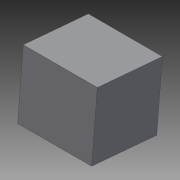
# Autodesk Inventor part: Part1
Saved by Autodesk Inventor 2014 SP2 (Build 180246200, 246)
## iProperties
Created: 2014-12-30
Part Number: Part1
Material: 一般
Document SubType Name: Modeling
Designer: hiratayuya
Density: 1 g/cm^3
Appearance: 既定
Author: hiratayuya
Autodesk Inventor part; units mm, degrees
ref_plane "YZ Plane" through (0, 0, 0) normal (1, 0, 0) x (0, 1, 0)
ref_plane "XZ Plane" through (0, 0, 0) normal (0, 1, 0) x (-1, 0, 0)
ref_plane "XY Plane" through (0, 0, 0) normal (0, 0, 1) x (1, 0, 0)
sketch "スケッチ1" plane through (0, 0, 0) normal (0, 1, 0) x (-1, 0, 0)
  line L0 (-7.5, -10) -> (7.5, -10)
  line L1 (7.5, -10) -> (7.5, 10)
  line L2 (7.5, 10) -> (-7.5, 10)
  line L3 (-7.5, 10) -> (-7.5, -10)
  line L4 (-7.5, -10) -> (7.5, 10) construction
  line L5 (7.5, -10) -> (-7.5, 10) construction
  line L6 (-7.5, 10) -> (7.5, 10)
  line L7 (7.5, 10) -> (7.5, 4)
  line L8 (7.5, 4) -> (-7.5, 4)
  line L9 (-7.5, 4) -> (-7.5, 10)
  line L10 (-7.5, -10) -> (7.5, -10)
  line L11 (7.5, -10) -> (7.5, -4)
  line L12 (7.5, -4) -> (-7.5, -4)
  line L13 (-7.5, -4) -> (-7.5, -10)
  point P0 (0, 0)
  dimension "d0" = 15
  dimension "d1" = 20
  dimension "d2" = 6
  dimension "d3" = 6
  constraints: 28 end point, 6 parallel, 3 horizontal, 3 perpendicular, 2 midpoint, 2 point on line
  measures "d0" distance of L1.end L2.end
  measures "d1" distance of L0.end L1.end
  measures "d2" distance between parallel lines of L8 L6
  measures "d3" distance between parallel lines of L10 L12
extrude "押し出し1" add sketch "スケッチ1" along normal blind 6 contours L3 L12 L1 L0 | L3 L2 L1 L8
sketch "スケッチ2" plane through (0, 6, 0) normal (0, 1, 0) x (1, 0, 0)
  line L0 (7.5, 10) -> (-7.5, 10) projected
  line L1 (-7.5, 10) -> (-7.5, 4) projected
  line L2 (-7.5, 4) -> (7.5, 4) projected
  line L3 (7.5, 4) -> (7.5, 10) projected
  line L4 (-7.5, -5.5) -> (7.5, -5.5)
  line L5 (7.5, -5.5) -> (7.5, 5.5)
  line L6 (7.5, 5.5) -> (-7.5, 5.5)
  line L7 (-7.5, 5.5) -> (-7.5, -5.5)
  line L8 (-7.5, -5.5) -> (7.5, 5.5) construction
  line L9 (7.5, -5.5) -> (-7.5, 5.5) construction
  point P0 (0, 0)
  dimension "d6" = 11
  constraints: 12 end point, 2 midpoint, 2 parallel, 1 horizontal, 1 perpendicular, 1 point on line
  measures "d6" distance between parallel lines of L4 L6
extrude "押し出し2" add sketch "スケッチ2" along normal blind 20 contours L3 L2 L1 L6 | L5 L4 L7 L2
sketch "スケッチ3" plane through (7.5, 0, -4) normal (1, 0, 0) x (0, 0, -1)
  line L0 (1.5, 6) -> (1.5, 26) projected
  line L1 (-9.5, 26) -> (1.5, 26) projected
  line L2 (-9.5, 26) -> (1.5, 25.0376)
  point P0 (-4, 0)
  dimension "d9" = 5
  constraints: 2 end point, 1 point on line
  measures "d9" angle of L1 L2
extrude "押し出し3" cut sketch "スケッチ3" against normal blind 20
sketch "スケッチ4" plane through (-7.5, 26, 5.5) normal (0, 0.9961947, -0.0871557) x (1, 0, 0)
  line L0 (0, 0) -> (0, 11.042) projected
  line L1 (0, 0) -> (15, 0) projected
  line L2 (15, 11.042) -> (15, 0) projected
  line L3 (0, 11.042) -> (15, 11.042) projected
  line L4 (-2, 13.042) -> (17, 13.042)
  line L5 (17, 13.042) -> (17, -2)
  line L6 (17, -2) -> (-2, -2)
  line L7 (-2, -2) -> (-2, 13.042)
  point P0 (7.5, 7.7451)
  dimension "d12" = 2
  dimension "d13" = 2
  dimension "d14" = 2
  dimension "d15" = 2
  constraints: 8 end point, 2 parallel, 1 horizontal, 1 perpendicular
  measures "d12" distance between parallel lines of L4 L3
  measures "d13" distance between parallel lines of L6 L1
  measures "d14" distance between parallel lines of L5 L2
  measures "d15" distance between parallel lines of L0 L7
extrude "押し出し4" add sketch "スケッチ4" along normal blind 15 contours L0 L3 L2 L1 | L4 L5 L6 L7
sketch "スケッチ5" plane through (9.5, 24.8633, -7.4924) normal (0, -0.0871557, -0.9961947) x (-1, 0, 0)
  line L0 (19, 0) -> (0, 0) projected
  line L1 (11.6915, 7.5253) -> (11.6915, 2.7045)
  line L2 (11.6915, 2.7045) -> (7.6915, 2.7045)
  line L3 (7.6915, 2.7045) -> (7.6915, 7.5253)
  line L4 (9.6915, 7.5253) -> (11.6915, 2.7045) construction
  line L5 (9.6915, 7.5253) -> (7.6915, 2.7045) construction
  line L6 (7.6915, 7.5253) -> (11.6915, 7.5253)
  line L7 (11.6915, 5.1149) -> (13.1915, 5.1149)
  line L8 (13.1915, 5.1149) -> (13.1915, 1.1149)
  line L9 (13.1915, 1.1149) -> (11.6915, 1.1149)
  line L10 (11.6915, 1.1149) -> (11.6915, 5.1149)
  line L11 (7.6915, 5.1149) -> (6.1915, 5.1149)
  line L12 (6.1915, 5.1149) -> (6.1915, 1.1149)
  line L13 (6.1915, 1.1149) -> (7.6915, 1.1149)
  line L14 (7.6915, 1.1149) -> (7.6915, 5.1149)
  line L15 (11.6915, 7.5253) -> (14.6915, 7.5253)
  line L16 (14.6915, 7.5253) -> (14.6915, 10.5253)
  line L17 (14.6915, 10.5253) -> (11.6915, 10.5253)
  line L18 (11.6915, 10.5253) -> (11.6915, 7.5253)
  line L19 (7.6915, 7.5253) -> (4.6915, 7.5253)
  line L20 (4.6915, 7.5253) -> (4.6915, 10.5253)
  line L21 (4.6915, 10.5253) -> (7.6915, 10.5253)
  line L22 (7.6915, 10.5253) -> (7.6915, 7.5253)
  point P0 (9.5, -25.4217)
  dimension "d18" = 4
  dimension "d19" = 1.5
  dimension "d20" = 4
  dimension "d21" = 1.5
  dimension "d22" = 3
  dimension "d23" = 3
  dimension "d24" = 3
  dimension "d25" = 2.7045
  constraints: 44 end point, 9 parallel, 4 horizontal, 4 perpendicular, 3 midpoint, 2 point on line
  measures "d18" distance of L3.end L1.start
  measures "d19" distance of L7.start L7.end
  measures "d20" distance of L7.end L8.end
  measures "d21" distance of L13.end L12.end
  measures "d22" distance of L17.end L16.end
  measures "d23" distance of L15.end L16.end
  measures "d24" distance of L20.end L21.end
  measures "d25" distance between parallel lines of L0 L2
extrude "押し出し5" cut sketch "スケッチ5" against normal blind 1
sketch "スケッチ6" plane through (7.5, 0, 10) normal (1, 0, 0) x (0, 0, -1)
  line L0 (4.5, 6) -> (4.5, 26) projected
  line L1 (0, 6) -> (4.5, 6) projected
  line L2 (0, 0) -> (0, 6) projected
  line L3 (0, 0) -> (6, 0) projected
  line L4 (6, 0) -> (6, 6) projected
  line L5 (6, 6) -> (14, 6) projected
  line L6 (14, 0) -> (14, 6) projected
  line L7 (14, 0) -> (20, 0) projected
  line L8 (20, 0) -> (20, 6) projected
  line L9 (15.5, 6) -> (20, 6) projected
  line L10 (15.5, 6) -> (15.5, 25.0376) projected
  line L11 (15.5, 25.0376) -> (4.5, 25.0376)
  point P0 (10, 0)
  constraints: 2 end point, 1 perpendicular, 1 point on line
extrude "押し出し6" cut sketch "スケッチ6" against normal blind 100
sketch "スケッチ7" plane through (-7.5, 25.0376, 5.5) normal (-1, 0, 0) x (0, 0, 1)
  line L0 (-11, 0) -> (0, 0) projected
  line L1 (0, 0) -> (0, 0.9624) projected
  line L2 (0, 0.9624) -> (-11, 0) projected
  point P0 (-5.5, -25.0376)
extrude "押し出し7" cut sketch "スケッチ7" against normal blind 100
sketch "スケッチ8" plane through (9.5, 24.8633, -7.4924) normal (0, -0.0871557, -0.9961947) x (-1, 0, 0)
  line L0 (19, 0) -> (0, 0) projected
  line L1 (19, 0) -> (19, 15) projected
  line L2 (0, 15) -> (19, 15) projected
  line L3 (0, 0) -> (0, 15) projected
  line L4 (1, 15) -> (1, 0)
  line L5 (18, 15) -> (18, 0)
  point P0 (9.5, -25.4217)
  dimension "d32" = 1
  dimension "d33" = 1
  constraints: 4 end point, 4 point on line, 2 perpendicular
  measures "d32" distance between parallel lines of L4 L3
  measures "d33" distance between parallel lines of L1 L5
extrude "押し出し8" cut sketch "スケッチ8" against normal blind 100 contours L0 L5 L2 L1 | L0 L3 L2 L4
